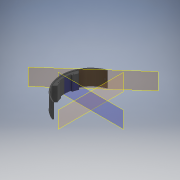
# Autodesk Inventor part: protect_v2
Saved by Autodesk Inventor 2020 (Build 240168000, 168)
## iProperties
Created: 2024-10-31
Part Number: protect_v2
Material: Типовые
Document SubType Name: Modeling
Designer: Ivan
Density: 0.80427 g/cm^3
Appearance: Типовые
Mass: 79 g
Surface Area: 341.156 cm^2
Volume: 98.2257 cm^3
Author: Ivan
Autodesk Inventor part; units mm, degrees
ref_plane "XZ Plane" through (0, 0, 0) normal (0, 1, 0) x (-1, 0, 0)
ref_plane "XY Plane" through (0, 0, 0) normal (0, 0, 1) x (1, 0, 0)
derived "floor_v2.ipt"
sketch "Эскиз2" plane through (0, 0, 0) normal (0, 1, 0) x (1, 0, 0)
  circle A0 centre (0, 0) radius 107.5
  circle A1 centre (0, 0) radius 104
  line L0 (0, 0) -> (104, 0) construction
  line L1 (0, 0) -> (0, -104) construction
  line L2 (0, 0) -> (-104, 0) construction
  line L3 (0, 0) -> (0, 104) construction
  line L4 (104, 0) -> (0, -104) construction
  line L5 (0, 104) -> (-104, 0) construction
  line L6 (0, -104) -> (-104, 0) construction
  line L7 (104, 0) -> (0, 104) construction
  line L8 (0, 0) -> (-73.5391, -73.5391) construction
  line L9 (0, 0) -> (73.5391, -73.5391) construction
  line L10 (0, 0) -> (73.5391, 73.5391) construction
  line L11 (0, 0) -> (-73.5391, 73.5391) construction
  line L12 (-38.4471, -82.2877) -> (-82.2877, -38.4471)
  line L13 (-38.4471, -82.2877) -> (-48.2758, -92.1165)
  line L14 (-82.2877, -38.4471) -> (-92.1165, -48.2758)
  line L15 (92.1165, -48.2758) -> (82.2877, -38.4471)
  line L16 (82.2877, -38.4471) -> (38.4471, -82.2877)
  line L17 (38.4471, -82.2877) -> (48.2758, -92.1165)
  line L18 (48.2758, 92.1165) -> (38.4471, 82.2877)
  line L19 (38.4471, 82.2877) -> (82.2877, 38.4471)
  line L20 (82.2877, 38.4471) -> (92.1165, 48.2758)
  line L21 (-48.2758, 92.1165) -> (-38.4471, 82.2877)
  line L22 (-38.4471, 82.2877) -> (-82.2877, 38.4471)
  line L23 (-82.2877, 38.4471) -> (-92.1165, 48.2758)
  line L24 (0, -107.5) -> (0, -79.5) construction
  circle A2 centre (0, -116.5) radius 37 construction
  circle A3 centre (0, -127) radius 47.5
  line L25 (0, 107.5) -> (0, 79.5) construction
  circle A4 centre (0, 127) radius 47.5
  line L26 (-92.1165, 48.2758) -> (-94.7051, 50.8645)
  line L27 (-48.2758, 92.1165) -> (-50.8645, 94.7051)
  line L28 (48.2758, 92.1165) -> (50.8645, 94.7051)
  line L29 (92.1165, 48.2758) -> (94.7051, 50.8645)
  line L30 (92.1165, -48.2758) -> (94.7051, -50.8645)
  line L31 (48.2758, -92.1165) -> (50.8645, -94.7051)
  line L32 (-92.1165, -48.2758) -> (-94.7051, -50.8645)
  line L33 (-48.2758, -92.1165) -> (-50.8645, -94.7051)
  point P0 (-52, -52)
  point P1 (-52, 52)
  point P2 (52, 52)
  point P3 (52, -52)
  point P4 (-60.3674, -60.3674)
  point P5 (60.3674, -60.3674)
  point P6 (60.3674, 60.3674)
  point P7 (-60.3674, 60.3674)
  point P8 (-36.9892, -97.1998)
  point P9 (36.9892, -97.1998)
  point P10 (36.9892, 97.1998)
  point P11 (-36.9892, 97.1998)
  point P12 (-39.1587, 100.1142)
  point P13 (-39.1587, -100.1142)
sketch "Эскиз7" plane through (0, 2, 0) normal (0, -1, 0) x (-1, 0, 0)
  circle A0 centre (0, 0) radius 94.2655 construction
  circle A1 centre (-90.3481, 26.8924) radius 1.5
  circle A2 centre (-90.3481, -26.8924) radius 1.5
  circle A3 centre (90.3481, 26.8924) radius 1.5
  circle A4 centre (90.3481, -26.8924) radius 1.5
  line L0 (-92.1165, 48.2758) -> (-82.2877, 38.4471)
  line L1 (-82.2877, -38.4471) -> (-92.1165, -48.2758)
  line L2 (92.1165, -48.2758) -> (82.2877, -38.4471)
  line L3 (82.2877, 38.4471) -> (92.1165, 48.2758)
sketch "Эскиз4" plane through (0, 0, 0) normal (0, 1, 0) x (-1, 0, 0)
  circle A0 centre (0, 0) radius 104 projected
  line L0 (92.1165, 48.2758) -> (82.2877, 38.4471) projected
  line L1 (82.2877, -38.4471) -> (92.1165, -48.2758) projected
  circle A1 centre (90.3481, -26.8924) radius 1.5 projected
  circle A2 centre (90.3481, 26.8924) radius 1.5 projected
  arc A3 (82.2877, -38.4471) -> (82.2877, 38.4471) centre (0, 0) ccw
  line L2 (90.3481, 26.8924) -> (0, 0) construction
  line L3 (0, 0) -> (90.3481, -26.8924) construction
  line L4 (90.3481, 26.8924) -> (91.7858, 27.3203) construction
  line L5 (90.3481, -26.8924) -> (91.7858, -27.3203) construction
  arc A4 (91.7858, -27.3203) -> (91.7858, 27.3203) centre (0, 0) ccw
  line L6 (88.5247, 20.3179) -> (93.3386, 21.4227)
  line L7 (88.5247, -20.3179) -> (93.3386, -21.4227)
  dimension "d1" = 6
  dimension "d2" = 6
  constraints: 12 end point, 8 point on circle, 2 centre point, 2 coincident, 2 collinear, 2 point on line, 4 other
  measures "d1" distance from line of L6 L2.start
  measures "d2" distance from line of L7 L3.end
extrude "Выдавливание1" add sketch "Эскиз4" along normal blind 51.15 contours A0 L1 A3 L7 A4 L6 L0
sketch "Эскиз5" plane through (0, 0, 0) normal (0, -1, 0) x (1, 0, 0)
  line L0 (-38.4471, 82.2877) -> (-48.2758, 92.1165) projected
  line L1 (-48.2758, -92.1165) -> (-38.4471, -82.2877) projected
  circle A0 centre (0, 0) radius 104 projected
  circle A1 centre (0, 0) radius 107.5 projected
  line L2 (-48.2758, 92.1165) -> (-50.8645, 94.7051)
  line L3 (-48.2758, -92.1165) -> (-50.8645, -94.7051)
  constraints: 4 end point, 2 collinear, 2 point on circle
extrude "Выдавливание2" add sketch "Эскиз2" along normal blind 53.15 and the other way blind 2 contours A4 A1 L27 A0 | A0 L33 A1 A3 | L27 A1 L26 A0 | A0 L32 A1 L33 | L26 A1 L32 A0
ref_plane "РабПлоскость1" through (-36.9892, 0, -97.1998) normal (0.6637718, 0, 0.7479351) x (0, 1, 0)
sketch "Эскиз6" plane through (-36.9892, 0, -97.1998) normal (0.6637718, 0, 0.7479351) x (0, 1, 0)
  line L0 (53.15, -0.3118) -> (-2, -0.3118) projected
  line L1 (-2, 0) -> (53.15, 0) projected
  line L2 (25.575, 0) -> (25.575, 67) construction
  circle A0 centre (25.575, 6.1895) radius 1.6
  point P0 (0, 36.853)
  dimension "d9" = 3.2
  dimension "d10" = 6.1895
  constraints: 2 end point, 1 centre point, 1 midpoint, 1 point on line, 1 vertical
  measures "d9" diameter of A0
  measures "d10" distance from line of L1 A0.centre
extrude "Выдавливание3" cut sketch "Эскиз6" against normal blind 10
chamfer "Фаска1" distance 1.4 angle 45 1 edges at (-45.4505, 23.975, -97.4192)
ref_plane "РабПлоскость2" through (0, 0, 0) normal (0, 0, -1) x (0, -1, 0)
mirror "Зеркальное отражение1" about plane through (0, 0, 0) normal (0, 0, -1) of "Выдавливание3", "Фаска1"
equation "\"d2\" = d1"
